Autodesk Fusion 360 part; units mm, degrees
(part 10 of 12)
  line L360 (-90.518, -7.747) -> (-90.518, -11.547)
  line L361 (-94.318, -11.547) -> (-94.318, -7.747)
  line L362 (-90.518, -11.547) -> (-94.318, -11.547)
  line L363 (-94.318, -7.747) -> (-90.518, -7.747)
  arc A1946 (-90.5461, -4.953) -> (-94.5339, -4.953) centre (-92.54, -4.953) ccw
  arc A1947 (-94.5339, -4.953) -> (-90.5461, -4.953) centre (-92.54, -4.953) ccw
  arc A1948 (-88.3109, -5.08) -> (-86.6091, -5.08) centre (-87.46, -5.08) ccw
  arc A1949 (-86.6091, -5.08) -> (-88.3109, -5.08) centre (-87.46, -5.08) ccw
  arc A1950 (-96.7691, -5.08) -> (-98.4709, -5.08) centre (-97.62, -5.08) ccw
  arc A1951 (-98.4709, -5.08) -> (-96.7691, -5.08) centre (-97.62, -5.08) ccw
  line L364 (-60.518, -11.547) -> (-64.318, -11.547)
  line L365 (-64.318, -7.747) -> (-60.518, -7.747)
  line L366 (-60.518, -7.747) -> (-60.518, -11.547)
  line L367 (-64.318, -11.547) -> (-64.318, -7.747)
  arc A1952 (-64.5339, -4.953) -> (-60.5461, -4.953) centre (-62.54, -4.953) ccw
  arc A1953 (-60.5461, -4.953) -> (-64.5339, -4.953) centre (-62.54, -4.953) ccw
  arc A1954 (-56.6091, -5.08) -> (-58.3109, -5.08) centre (-57.46, -5.08) ccw
  arc A1955 (-58.3109, -5.08) -> (-56.6091, -5.08) centre (-57.46, -5.08) ccw
  arc A1956 (-66.7691, -5.08) -> (-68.4709, -5.08) centre (-67.62, -5.08) ccw
  arc A1957 (-68.4709, -5.08) -> (-66.7691, -5.08) centre (-67.62, -5.08) ccw
  line L368 (-34.318, -7.747) -> (-30.518, -7.747)
  line L369 (-30.518, -11.547) -> (-34.318, -11.547)
  line L370 (-30.518, -7.747) -> (-30.518, -11.547)
  line L371 (-34.318, -11.547) -> (-34.318, -7.747)
  arc A1958 (-30.5461, -4.953) -> (-34.5339, -4.953) centre (-32.54, -4.953) ccw
  arc A1959 (-34.5339, -4.953) -> (-30.5461, -4.953) centre (-32.54, -4.953) ccw
  arc A1960 (-26.6091, -5.08) -> (-28.3109, -5.08) centre (-27.46, -5.08) ccw
  arc A1961 (-28.3109, -5.08) -> (-26.6091, -5.08) centre (-27.46, -5.08) ccw
  arc A1962 (-36.7691, -5.08) -> (-38.4709, -5.08) centre (-37.62, -5.08) ccw
  arc A1963 (-38.4709, -5.08) -> (-36.7691, -5.08) centre (-37.62, -5.08) ccw
  line L372 (10.033, -11.801) -> (10.033, -8.001)
  line L373 (13.833, -11.801) -> (10.033, -11.801)
  line L374 (13.833, -8.001) -> (13.833, -11.801)
  line L375 (10.033, -8.001) -> (13.833, -8.001)
  arc A1964 (9.8171, -5.207) -> (13.8049, -5.207) centre (11.811, -5.207) ccw
  arc A1965 (13.8049, -5.207) -> (9.8171, -5.207) centre (11.811, -5.207) ccw
  arc A1966 (17.7419, -5.334) -> (16.0401, -5.334) centre (16.891, -5.334) ccw
  arc A1967 (16.0401, -5.334) -> (17.7419, -5.334) centre (16.891, -5.334) ccw
  arc A1968 (7.5819, -5.334) -> (5.8801, -5.334) centre (6.731, -5.334) ccw
  arc A1969 (5.8801, -5.334) -> (7.5819, -5.334) centre (6.731, -5.334) ccw
  line L376 (49.1491, -12.055) -> (49.1491, -8.255)
  line L377 (49.1491, -8.255) -> (52.9491, -8.255)
  line L378 (52.9491, -8.255) -> (52.9491, -12.055)
  line L379 (52.9491, -12.055) -> (49.1491, -12.055)
  arc A1970 (52.921, -5.461) -> (48.9332, -5.461) centre (50.9271, -5.461) ccw
  arc A1971 (48.9332, -5.461) -> (52.921, -5.461) centre (50.9271, -5.461) ccw
  arc A1972 (55.1562, -5.588) -> (56.858, -5.588) centre (56.0071, -5.588) ccw
  arc A1973 (56.858, -5.588) -> (55.1562, -5.588) centre (56.0071, -5.588) ccw
  arc A1974 (46.698, -5.588) -> (44.9962, -5.588) centre (45.8471, -5.588) ccw
  arc A1975 (44.9962, -5.588) -> (46.698, -5.588) centre (45.8471, -5.588) ccw
  line L380 (-196.538, -36.3221) -> (-192.738, -36.3221)
  line L381 (-192.738, -36.3221) -> (-192.738, -40.1221)
  line L382 (-196.538, -40.1221) -> (-196.538, -36.3221)
  line L383 (-192.738, -40.1221) -> (-196.538, -40.1221)
  arc A1976 (-192.7661, -33.5281) -> (-196.7539, -33.5281) centre (-194.76, -33.5281) ccw
  arc A1977 (-196.7539, -33.5281) -> (-192.7661, -33.5281) centre (-194.76, -33.5281) ccw
  arc A1978 (-188.8291, -33.6551) -> (-190.5309, -33.6551) centre (-189.68, -33.6551) ccw
  arc A1979 (-190.5309, -33.6551) -> (-188.8291, -33.6551) centre (-189.68, -33.6551) ccw
  arc A1980 (-198.9891, -33.6551) -> (-200.6909, -33.6551) centre (-199.84, -33.6551) ccw
  arc A1981 (-200.6909, -33.6551) -> (-198.9891, -33.6551) centre (-199.84, -33.6551) ccw
  line L384 (-162.738, -36.3221) -> (-162.738, -40.1221)
  line L385 (-166.538, -36.3221) -> (-162.738, -36.3221)
  line L386 (-162.738, -40.1221) -> (-166.538, -40.1221)
  line L387 (-166.538, -40.1221) -> (-166.538, -36.3221)
  arc A1982 (-162.7661, -33.5281) -> (-166.7539, -33.5281) centre (-164.76, -33.5281) ccw
  arc A1983 (-166.7539, -33.5281) -> (-162.7661, -33.5281) centre (-164.76, -33.5281) ccw
  arc A1984 (-158.8291, -33.6551) -> (-160.5309, -33.6551) centre (-159.68, -33.6551) ccw
  arc A1985 (-160.5309, -33.6551) -> (-158.8291, -33.6551) centre (-159.68, -33.6551) ccw
  arc A1986 (-168.9891, -33.6551) -> (-170.6909, -33.6551) centre (-169.84, -33.6551) ccw
  arc A1987 (-170.6909, -33.6551) -> (-168.9891, -33.6551) centre (-169.84, -33.6551) ccw
  line L388 (-132.738, -40.1221) -> (-136.538, -40.1221)
  line L389 (-136.538, -36.3221) -> (-132.738, -36.3221)
  line L390 (-136.538, -40.1221) -> (-136.538, -36.3221)
  line L391 (-132.738, -36.3221) -> (-132.738, -40.1221)
  arc A1988 (-132.7661, -33.5281) -> (-136.7539, -33.5281) centre (-134.76, -33.5281) ccw
  arc A1989 (-136.7539, -33.5281) -> (-132.7661, -33.5281) centre (-134.76, -33.5281) ccw
  arc A1990 (-128.8291, -33.6551) -> (-130.5309, -33.6551) centre (-129.68, -33.6551) ccw
  arc A1991 (-130.5309, -33.6551) -> (-128.8291, -33.6551) centre (-129.68, -33.6551) ccw
  arc A1992 (-140.6909, -33.6551) -> (-138.9891, -33.6551) centre (-139.84, -33.6551) ccw
  arc A1993 (-138.9891, -33.6551) -> (-140.6909, -33.6551) centre (-139.84, -33.6551) ccw
  line L392 (-102.738, -36.3221) -> (-102.738, -40.1221)
  line L393 (-106.538, -40.1221) -> (-106.538, -36.3221)
  line L394 (-102.738, -40.1221) -> (-106.538, -40.1221)
  line L395 (-106.538, -36.3221) -> (-102.738, -36.3221)
  arc A1994 (-102.7661, -33.5281) -> (-106.7539, -33.5281) centre (-104.76, -33.5281) ccw
  arc A1995 (-106.7539, -33.5281) -> (-102.7661, -33.5281) centre (-104.76, -33.5281) ccw
  arc A1996 (-98.8291, -33.6551) -> (-100.5309, -33.6551) centre (-99.68, -33.6551) ccw
  arc A1997 (-100.5309, -33.6551) -> (-98.8291, -33.6551) centre (-99.68, -33.6551) ccw
  arc A1998 (-108.9891, -33.6551) -> (-110.6909, -33.6551) centre (-109.84, -33.6551) ccw
  arc A1999 (-110.6909, -33.6551) -> (-108.9891, -33.6551) centre (-109.84, -33.6551) ccw
  line L396 (-76.538, -40.1221) -> (-76.538, -36.3221)
  line L397 (-76.538, -36.3221) -> (-72.738, -36.3221)
  line L398 (-72.738, -36.3221) -> (-72.738, -40.1221)
  line L399 (-72.738, -40.1221) -> (-76.538, -40.1221)
  arc A2000 (-76.7539, -33.5281) -> (-72.7661, -33.5281) centre (-74.76, -33.5281) ccw
  arc A2001 (-72.7661, -33.5281) -> (-76.7539, -33.5281) centre (-74.76, -33.5281) ccw
  arc A2002 (-68.8291, -33.6551) -> (-70.5309, -33.6551) centre (-69.68, -33.6551) ccw
  arc A2003 (-70.5309, -33.6551) -> (-68.8291, -33.6551) centre (-69.68, -33.6551) ccw
  arc A2004 (-80.6909, -33.6551) -> (-78.9891, -33.6551) centre (-79.84, -33.6551) ccw
  arc A2005 (-78.9891, -33.6551) -> (-80.6909, -33.6551) centre (-79.84, -33.6551) ccw
  line L400 (-42.738, -40.1221) -> (-46.538, -40.1221)
  line L401 (-46.538, -36.3221) -> (-42.738, -36.3221)
  line L402 (-42.738, -36.3221) -> (-42.738, -40.1221)
  line L403 (-46.538, -40.1221) -> (-46.538, -36.3221)
  arc A2006 (-46.7539, -33.5281) -> (-42.7661, -33.5281) centre (-44.76, -33.5281) ccw
  arc A2007 (-42.7661, -33.5281) -> (-46.7539, -33.5281) centre (-44.76, -33.5281) ccw
  arc A2008 (-40.5309, -33.6551) -> (-38.8291, -33.6551) centre (-39.68, -33.6551) ccw
  arc A2009 (-38.8291, -33.6551) -> (-40.5309, -33.6551) centre (-39.68, -33.6551) ccw
  arc A2010 (-48.9891, -33.6551) -> (-50.6909, -33.6551) centre (-49.84, -33.6551) ccw
  arc A2011 (-50.6909, -33.6551) -> (-48.9891, -33.6551) centre (-49.84, -33.6551) ccw
  line L404 (-12.738, -40.1221) -> (-16.538, -40.1221)
  line L405 (-12.738, -36.3221) -> (-12.738, -40.1221)
  line L406 (-16.538, -40.1221) -> (-16.538, -36.3221)
  line L407 (-16.538, -36.3221) -> (-12.738, -36.3221)
  arc A2012 (-16.7539, -33.5281) -> (-12.7661, -33.5281) centre (-14.76, -33.5281) ccw
  arc A2013 (-12.7661, -33.5281) -> (-16.7539, -33.5281) centre (-14.76, -33.5281) ccw
  line L408 (-12.7661, -33.5281) -> (-12.7661, -33.5281)
  arc A2014 (-8.8291, -33.6551) -> (-10.5309, -33.6551) centre (-9.68, -33.6551) ccw
  arc A2015 (-10.5309, -33.6551) -> (-8.8291, -33.6551) centre (-9.68, -33.6551) ccw
  arc A2016 (-20.6909, -33.6551) -> (-18.9891, -33.6551) centre (-19.84, -33.6551) ccw
  arc A2017 (-18.9891, -33.6551) -> (-20.6909, -33.6551) centre (-19.84, -33.6551) ccw
  line L409 (17.262, -36.3221) -> (17.262, -40.1221)
  line L410 (13.462, -36.3221) -> (17.262, -36.3221)
  line L411 (13.462, -40.1221) -> (13.462, -36.3221)
  line L412 (17.262, -40.1221) -> (13.462, -40.1221)
  arc A2018 (13.2461, -33.5281) -> (17.2339, -33.5281) centre (15.24, -33.5281) ccw
  arc A2019 (17.2339, -33.5281) -> (13.2461, -33.5281) centre (15.24, -33.5281) ccw
  line L413 (17.2339, -33.5281) -> (17.2339, -33.5281)
  arc A2020 (21.1709, -33.6551) -> (19.4691, -33.6551) centre (20.32, -33.6551) ccw
  arc A2021 (19.4691, -33.6551) -> (21.1709, -33.6551) centre (20.32, -33.6551) ccw
  arc A2022 (11.0109, -33.6551) -> (9.3091, -33.6551) centre (10.16, -33.6551) ccw
  arc A2023 (9.3091, -33.6551) -> (11.0109, -33.6551) centre (10.16, -33.6551) ccw
  line L414 (49.1466, -41.1381) -> (49.1466, -37.3381)
  line L415 (52.9466, -37.3381) -> (52.9466, -41.1381)
  line L416 (49.1466, -37.3381) -> (52.9466, -37.3381)
  line L417 (52.9466, -41.1381) -> (49.1466, -41.1381)
  arc A2024 (48.9307, -34.5441) -> (52.9185, -34.5441) centre (50.9246, -34.5441) ccw
  arc A2025 (52.9185, -34.5441) -> (48.9307, -34.5441) centre (50.9246, -34.5441) ccw
  arc A2026 (56.8555, -34.6711) -> (55.1537, -34.6711) centre (56.0046, -34.6711) ccw
  arc A2027 (55.1537, -34.6711) -> (56.8555, -34.6711) centre (56.0046, -34.6711) ccw
  arc A2028 (44.9937, -34.6711) -> (46.6955, -34.6711) centre (45.8446, -34.6711) ccw
  arc A2029 (46.6955, -34.6711) -> (44.9937, -34.6711) centre (45.8446, -34.6711) ccw
  line L418 (-185.9511, -63.3791) -> (-185.9511, -67.1791)
  line L419 (-185.9511, -67.1791) -> (-189.7511, -67.1791)
  line L420 (-189.7511, -63.3791) -> (-185.9511, -63.3791)
  line L421 (-189.7511, -67.1791) -> (-189.7511, -63.3791)
  arc A2030 (-189.967, -60.5851) -> (-185.9792, -60.5851) centre (-187.9731, -60.5851) ccw
  arc A2031 (-185.9792, -60.5851) -> (-189.967, -60.5851) centre (-187.9731, -60.5851) ccw
  arc A2032 (-182.0422, -60.7121) -> (-183.744, -60.7121) centre (-182.8931, -60.7121) ccw
  arc A2033 (-183.744, -60.7121) -> (-182.0422, -60.7121) centre (-182.8931, -60.7121) ccw
  arc A2034 (-192.2022, -60.7121) -> (-193.904, -60.7121) centre (-193.0531, -60.7121) ccw
  arc A2035 (-193.904, -60.7121) -> (-192.2022, -60.7121) centre (-193.0531, -60.7121) ccw
  line L422 (-155.9511, -67.1791) -> (-159.7511, -67.1791)
  line L423 (-155.9511, -63.3791) -> (-155.9511, -67.1791)
  line L424 (-159.7511, -63.3791) -> (-155.9511, -63.3791)
  line L425 (-159.7511, -67.1791) -> (-159.7511, -63.3791)
  arc A2036 (-155.9792, -60.5851) -> (-159.967, -60.5851) centre (-157.9731, -60.5851) ccw
  arc A2037 (-159.967, -60.5851) -> (-155.9792, -60.5851) centre (-157.9731, -60.5851) ccw
  arc A2038 (-152.0422, -60.7121) -> (-153.744, -60.7121) centre (-152.8931, -60.7121) ccw
  arc A2039 (-153.744, -60.7121) -> (-152.0422, -60.7121) centre (-152.8931, -60.7121) ccw
  arc A2040 (-162.2022, -60.7121) -> (-163.904, -60.7121) centre (-163.0531, -60.7121) ccw
  arc A2041 (-163.904, -60.7121) -> (-162.2022, -60.7121) centre (-163.0531, -60.7121) ccw
  line L426 (-129.7511, -67.1791) -> (-129.7511, -63.3791)
  line L427 (-125.9511, -63.3791) -> (-125.9511, -67.1791)
  line L428 (-125.9511, -67.1791) -> (-129.7511, -67.1791)
  line L429 (-129.7511, -63.3791) -> (-125.9511, -63.3791)
  arc A2042 (-129.967, -60.5851) -> (-125.9792, -60.5851) centre (-127.9731, -60.5851) ccw
  arc A2043 (-125.9792, -60.5851) -> (-129.967, -60.5851) centre (-127.9731, -60.5851) ccw
  arc A2044 (-123.744, -60.7121) -> (-122.0422, -60.7121) centre (-122.8931, -60.7121) ccw
  arc A2045 (-122.0422, -60.7121) -> (-123.744, -60.7121) centre (-122.8931, -60.7121) ccw
  arc A2046 (-133.904, -60.7121) -> (-132.2022, -60.7121) centre (-133.0531, -60.7121) ccw
  arc A2047 (-132.2022, -60.7121) -> (-133.904, -60.7121) centre (-133.0531, -60.7121) ccw
  line L430 (-95.9511, -67.1791) -> (-99.7511, -67.1791)
  line L431 (-99.7511, -67.1791) -> (-99.7511, -63.3791)
  line L432 (-95.9511, -63.3791) -> (-95.9511, -67.1791)
  line L433 (-99.7511, -63.3791) -> (-95.9511, -63.3791)
  arc A2048 (-95.9792, -60.5851) -> (-99.967, -60.5851) centre (-97.9731, -60.5851) ccw
  arc A2049 (-99.967, -60.5851) -> (-95.9792, -60.5851) centre (-97.9731, -60.5851) ccw
  arc A2050 (-93.744, -60.7121) -> (-92.0422, -60.7121) centre (-92.8931, -60.7121) ccw
  arc A2051 (-92.0422, -60.7121) -> (-93.744, -60.7121) centre (-92.8931, -60.7121) ccw
  arc A2052 (-103.904, -60.7121) -> (-102.2022, -60.7121) centre (-103.0531, -60.7121) ccw
  arc A2053 (-102.2022, -60.7121) -> (-103.904, -60.7121) centre (-103.0531, -60.7121) ccw
  line L434 (-65.9511, -63.3791) -> (-65.9511, -67.1791)
  line L435 (-65.9511, -67.1791) -> (-69.7511, -67.1791)
  line L436 (-69.7511, -67.1791) -> (-69.7511, -63.3791)
  line L437 (-69.7511, -63.3791) -> (-65.9511, -63.3791)
  arc A2054 (-65.9792, -60.5851) -> (-69.967, -60.5851) centre (-67.9731, -60.5851) ccw
  arc A2055 (-69.967, -60.5851) -> (-65.9792, -60.5851) centre (-67.9731, -60.5851) ccw
  arc A2056 (-63.744, -60.7121) -> (-62.0422, -60.7121) centre (-62.8931, -60.7121) ccw
  arc A2057 (-62.0422, -60.7121) -> (-63.744, -60.7121) centre (-62.8931, -60.7121) ccw
  arc A2058 (-73.904, -60.7121) -> (-72.2022, -60.7121) centre (-73.0531, -60.7121) ccw
  arc A2059 (-72.2022, -60.7121) -> (-73.904, -60.7121) centre (-73.0531, -60.7121) ccw
  line L438 (-39.7511, -63.3791) -> (-35.9511, -63.3791)
  line L439 (-35.9511, -67.1791) -> (-39.7511, -67.1791)
  line L440 (-39.7511, -67.1791) -> (-39.7511, -63.3791)
  line L441 (-35.9511, -63.3791) -> (-35.9511, -67.1791)
  arc A2060 (-35.9792, -60.5851) -> (-39.967, -60.5851) centre (-37.9731, -60.5851) ccw
  arc A2061 (-39.967, -60.5851) -> (-35.9792, -60.5851) centre (-37.9731, -60.5851) ccw
  arc A2062 (-33.744, -60.7121) -> (-32.0422, -60.7121) centre (-32.8931, -60.7121) ccw
  arc A2063 (-32.0422, -60.7121) -> (-33.744, -60.7121) centre (-32.8931, -60.7121) ccw
  arc A2064 (-43.904, -60.7121) -> (-42.2022, -60.7121) centre (-43.0531, -60.7121) ccw
  arc A2065 (-42.2022, -60.7121) -> (-43.904, -60.7121) centre (-43.0531, -60.7121) ccw
  line L442 (3.175, -68.1891) -> (3.175, -64.3891)
  line L443 (6.975, -68.1891) -> (3.175, -68.1891)
  line L444 (6.975, -64.3891) -> (6.975, -68.1891)
  line L445 (3.175, -64.3891) -> (6.975, -64.3891)
  arc A2066 (6.9469, -61.5951) -> (2.9591, -61.5951) centre (4.953, -61.5951) ccw
  arc A2067 (2.9591, -61.5951) -> (6.9469, -61.5951) centre (4.953, -61.5951) ccw
  arc A2068 (9.1821, -61.7221) -> (10.8839, -61.7221) centre (10.033, -61.7221) ccw
  arc A2069 (10.8839, -61.7221) -> (9.1821, -61.7221) centre (10.033, -61.7221) ccw
  arc A2070 (0.7239, -61.7221) -> (-0.9779, -61.7221) centre (-0.127, -61.7221) ccw
  arc A2071 (-0.9779, -61.7221) -> (0.7239, -61.7221) centre (-0.127, -61.7221) ccw
  line L446 (-178.4989, -94.4882) -> (-174.6989, -94.4882)
  line L447 (-174.6989, -98.2882) -> (-178.4989, -98.2882)
  line L448 (-178.4989, -98.2882) -> (-178.4989, -94.4882)
  line L449 (-174.6989, -94.4882) -> (-174.6989, -98.2882)
  arc A2072 (-174.7269, -91.6942) -> (-178.7148, -91.6942) centre (-176.7209, -91.6942) ccw
  arc A2073 (-178.7148, -91.6942) -> (-174.7269, -91.6942) centre (-176.7209, -91.6942) ccw
  arc A2074 (-172.4917, -91.8212) -> (-170.7899, -91.8212) centre (-171.6408, -91.8212) ccw
  arc A2075 (-170.7899, -91.8212) -> (-172.4917, -91.8212) centre (-171.6408, -91.8212) ccw
  arc A2076 (-180.95, -91.8212) -> (-182.6518, -91.8212) centre (-181.8009, -91.8212) ccw
  arc A2077 (-182.6518, -91.8212) -> (-180.95, -91.8212) centre (-181.8009, -91.8212) ccw
  line L450 (55.8701, -71.7551) -> (55.8701, -75.5551)
  line L451 (52.0701, -75.5551) -> (52.0701, -71.7551)
  line L452 (52.0701, -71.7551) -> (55.8701, -71.7551)
  line L453 (55.8701, -75.5551) -> (52.0701, -75.5551)
  arc A2078 (51.8542, -68.9611) -> (55.842, -68.9611) centre (53.8481, -68.9611) ccw
  arc A2079 (55.842, -68.9611) -> (51.8542, -68.9611) centre (53.8481, -68.9611) ccw
  arc A2080 (58.0772, -69.0881) -> (59.779, -69.0881) centre (58.9281, -69.0881) ccw
  arc A2081 (59.779, -69.0881) -> (58.0772, -69.0881) centre (58.9281, -69.0881) ccw
  arc A2082 (47.9172, -69.0881) -> (49.619, -69.0881) centre (48.7681, -69.0881) ccw
  arc A2083 (49.619, -69.0881) -> (47.9172, -69.0881) centre (48.7681, -69.0881) ccw
  line L454 (-144.2823, -94.4882) -> (-144.2823, -98.2882)
  line L455 (-148.0823, -98.2882) -> (-148.0823, -94.4882)
  line L456 (-148.0823, -94.4882) -> (-144.2823, -94.4882)
  line L457 (-144.2823, -98.2882) -> (-148.0823, -98.2882)
  arc A2084 (-144.3104, -91.6942) -> (-148.2982, -91.6942) centre (-146.3043, -91.6942) ccw
  arc A2085 (-148.2982, -91.6942) -> (-144.3104, -91.6942) centre (-146.3043, -91.6942) ccw
  arc A2086 (-140.3734, -91.8212) -> (-142.0752, -91.8212) centre (-141.2243, -91.8212) ccw
  arc A2087 (-142.0752, -91.8212) -> (-140.3734, -91.8212) centre (-141.2243, -91.8212) ccw
  arc A2088 (-150.5335, -91.8212) -> (-152.2353, -91.8212) centre (-151.3844, -91.8212) ccw
  arc A2089 (-152.2353, -91.8212) -> (-150.5335, -91.8212) centre (-151.3844, -91.8212) ccw
  line L458 (-117.6658, -98.2882) -> (-117.6658, -94.4882)
  line L459 (-113.8658, -94.4882) -> (-113.8658, -98.2882)
  line L460 (-113.8658, -98.2882) -> (-117.6658, -98.2882)
  line L461 (-117.6658, -94.4882) -> (-113.8658, -94.4882)
  arc A2090 (-113.8939, -91.6942) -> (-117.8817, -91.6942) centre (-115.8878, -91.6942) ccw
  arc A2091 (-117.8817, -91.6942) -> (-113.8939, -91.6942) centre (-115.8878, -91.6942) ccw
  arc A2092 (-111.6587, -91.8212) -> (-109.9569, -91.8212) centre (-110.8078, -91.8212) ccw
  arc A2093 (-109.9569, -91.8212) -> (-111.6587, -91.8212) centre (-110.8078, -91.8212) ccw
  arc A2094 (-120.1169, -91.8212) -> (-121.8187, -91.8212) centre (-120.9678, -91.8212) ccw
  arc A2095 (-121.8187, -91.8212) -> (-120.1169, -91.8212) centre (-120.9678, -91.8212) ccw
  line L462 (-87.2492, -98.2882) -> (-87.2492, -94.4882)
  line L463 (-83.4492, -94.4882) -> (-83.4492, -98.2882)
  line L464 (-83.4492, -98.2882) -> (-87.2492, -98.2882)
  line L465 (-87.2492, -94.4882) -> (-83.4492, -94.4882)
  arc A2096 (-87.4651, -91.6942) -> (-83.4773, -91.6942) centre (-85.4712, -91.6942) ccw
  arc A2097 (-83.4773, -91.6942) -> (-87.4651, -91.6942) centre (-85.4712, -91.6942) ccw
  arc A2098 (-79.5403, -91.8212) -> (-81.2421, -91.8212) centre (-80.3912, -91.8212) ccw
  arc A2099 (-81.2421, -91.8212) -> (-79.5403, -91.8212) centre (-80.3912, -91.8212) ccw
  arc A2100 (-91.4021, -91.8212) -> (-89.7003, -91.8212) centre (-90.5512, -91.8212) ccw
  arc A2101 (-89.7003, -91.8212) -> (-91.4021, -91.8212) centre (-90.5512, -91.8212) ccw
  line L466 (-53.0326, -94.4882) -> (-53.0326, -98.2882)
  line L467 (-56.8326, -94.4882) -> (-53.0326, -94.4882)
  line L468 (-56.8326, -98.2882) -> (-56.8326, -94.4882)
  line L469 (-53.0326, -98.2882) -> (-56.8326, -98.2882)
  arc A2102 (-53.0607, -91.6942) -> (-57.0485, -91.6942) centre (-55.0546, -91.6942) ccw
  arc A2103 (-57.0485, -91.6942) -> (-53.0607, -91.6942) centre (-55.0546, -91.6942) ccw
  arc A2104 (-50.8255, -91.8212) -> (-49.1237, -91.8212) centre (-49.9746, -91.8212) ccw
  arc A2105 (-49.1237, -91.8212) -> (-50.8255, -91.8212) centre (-49.9746, -91.8212) ccw
  arc A2106 (-60.9855, -91.8212) -> (-59.2837, -91.8212) centre (-60.1346, -91.8212) ccw
  arc A2107 (-59.2837, -91.8212) -> (-60.9855, -91.8212) centre (-60.1346, -91.8212) ccw
  line L470 (-22.6161, -94.4882) -> (-22.6161, -98.2882)
  line L471 (-26.4161, -94.4882) -> (-22.6161, -94.4882)
  line L472 (-26.4161, -98.2882) -> (-26.4161, -94.4882)
  line L473 (-22.6161, -98.2882) -> (-26.4161, -98.2882)
  arc A2108 (-26.632, -91.6942) -> (-22.6441, -91.6942) centre (-24.638, -91.6942) ccw
  arc A2109 (-22.6441, -91.6942) -> (-26.632, -91.6942) centre (-24.638, -91.6942) ccw
  arc A2110 (-18.7071, -91.8212) -> (-20.4089, -91.8212) centre (-19.558, -91.8212) ccw
  arc A2111 (-20.4089, -91.8212) -> (-18.7071, -91.8212) centre (-19.558, -91.8212) ccw
  arc A2112 (-30.569, -91.8212) -> (-28.8672, -91.8212) centre (-29.7181, -91.8212) ccw
  arc A2113 (-28.8672, -91.8212) -> (-30.569, -91.8212) centre (-29.7181, -91.8212) ccw
  line L474 (3.937, -94.5894) -> (7.737, -94.5894)
  line L475 (3.937, -98.3894) -> (3.937, -94.5894)
  line L476 (7.737, -98.3894) -> (3.937, -98.3894)
  line L477 (7.737, -94.5894) -> (7.737, -98.3894)
  arc A2114 (7.7089, -91.7954) -> (3.7211, -91.7954) centre (5.715, -91.7954) ccw
  arc A2115 (3.7211, -91.7954) -> (7.7089, -91.7954) centre (5.715, -91.7954) ccw
  arc A2116 (11.6459, -91.9224) -> (9.9441, -91.9224) centre (10.795, -91.9224) ccw
  arc A2117 (9.9441, -91.9224) -> (11.6459, -91.9224) centre (10.795, -91.9224) ccw
  arc A2118 (-0.2159, -91.9224) -> (1.4859, -91.9224) centre (0.635, -91.9224) ccw
  arc A2119 (1.4859, -91.9224) -> (-0.2159, -91.9224) centre (0.635, -91.9224) ccw
  line L478 (-159.0293, -128.7242) -> (-159.0293, -124.9242)
  line L479 (-155.2293, -124.9242) -> (-155.2293, -128.7242)
  line L480 (-159.0293, -124.9242) -> (-155.2293, -124.9242)
  line L481 (-155.2293, -128.7242) -> (-159.0293, -128.7242)
  arc A2120 (-159.2452, -122.1302) -> (-155.2574, -122.1302) centre (-157.2513, -122.1302) ccw
  arc A2121 (-155.2574, -122.1302) -> (-159.2452, -122.1302) centre (-157.2513, -122.1302) ccw
  arc A2122 (-153.0222, -122.2572) -> (-151.3204, -122.2572) centre (-152.1713, -122.2572) ccw
  arc A2123 (-151.3204, -122.2572) -> (-153.0222, -122.2572) centre (-152.1713, -122.2572) ccw
  arc A2124 (-163.1822, -122.2572) -> (-161.4804, -122.2572) centre (-162.3313, -122.2572) ccw
  arc A2125 (-161.4804, -122.2572) -> (-163.1822, -122.2572) centre (-162.3313, -122.2572) ccw
  line L482 (-112.57, -128.7242) -> (-116.37, -128.7242)
  line L483 (-112.57, -124.9242) -> (-112.57, -128.7242)
  line L484 (-116.37, -124.9242) -> (-112.57, -124.9242)
  line L485 (-116.37, -128.7242) -> (-116.37, -124.9242)
  arc A2126 (-112.598, -122.1302) -> (-116.5859, -122.1302) centre (-114.5919, -122.1302) ccw
  arc A2127 (-116.5859, -122.1302) -> (-112.598, -122.1302) centre (-114.5919, -122.1302) ccw
  arc A2128 (-110.3628, -122.2572) -> (-108.661, -122.2572) centre (-109.5119, -122.2572) ccw
  arc A2129 (-108.661, -122.2572) -> (-110.3628, -122.2572) centre (-109.5119, -122.2572) ccw
  arc A2130 (-120.5229, -122.2572) -> (-118.8211, -122.2572) centre (-119.672, -122.2572) ccw
  arc A2131 (-118.8211, -122.2572) -> (-120.5229, -122.2572) centre (-119.672, -122.2572) ccw
  line L486 (-86.37, -128.7242) -> (-86.37, -124.9242)
  line L487 (-82.57, -128.7242) -> (-86.37, -128.7242)
  line L488 (-82.57, -124.9242) -> (-82.57, -128.7242)
  line L489 (-86.37, -124.9242) -> (-82.57, -124.9242)
  arc A2132 (-82.598, -122.1302) -> (-86.5859, -122.1302) centre (-84.5919, -122.1302) ccw
  arc A2133 (-86.5859, -122.1302) -> (-82.598, -122.1302) centre (-84.5919, -122.1302) ccw
  arc A2134 (-80.3628, -122.2572) -> (-78.661, -122.2572) centre (-79.5119, -122.2572) ccw
  arc A2135 (-78.661, -122.2572) -> (-80.3628, -122.2572) centre (-79.5119, -122.2572) ccw
  arc A2136 (-88.8211, -122.2572) -> (-90.5229, -122.2572) centre (-89.672, -122.2572) ccw
  arc A2137 (-90.5229, -122.2572) -> (-88.8211, -122.2572) centre (-89.672, -122.2572) ccw
  line L490 (-56.37, -128.7242) -> (-56.37, -124.9242)
  line L491 (-56.37, -124.9242) -> (-52.57, -124.9242)
  line L492 (-52.57, -128.7242) -> (-56.37, -128.7242)
  line L493 (-52.57, -124.9242) -> (-52.57, -128.7242)
  arc A2138 (-56.5859, -122.1302) -> (-52.598, -122.1302) centre (-54.5919, -122.1302) ccw
  arc A2139 (-52.598, -122.1302) -> (-56.5859, -122.1302) centre (-54.5919, -122.1302) ccw
  arc A2140 (-48.661, -122.2572) -> (-50.3628, -122.2572) centre (-49.5119, -122.2572) ccw
  arc A2141 (-50.3628, -122.2572) -> (-48.661, -122.2572) centre (-49.5119, -122.2572) ccw
  arc A2142 (-60.5229, -122.2572) -> (-58.8211, -122.2572) centre (-59.672, -122.2572) ccw
  arc A2143 (-58.8211, -122.2572) -> (-60.5229, -122.2572) centre (-59.672, -122.2572) ccw
  line L494 (-22.57, -124.9242) -> (-22.57, -128.7242)
  line L495 (-26.37, -124.9242) -> (-22.57, -124.9242)
  line L496 (-22.57, -128.7242) -> (-26.37, -128.7242)
  line L497 (-26.37, -128.7242) -> (-26.37, -124.9242)
  arc A2144 (-26.5859, -122.1302) -> (-22.598, -122.1302) centre (-24.5919, -122.1302) ccw
  arc A2145 (-22.598, -122.1302) -> (-26.5859, -122.1302) centre (-24.5919, -122.1302) ccw
  arc A2146 (-20.3628, -122.2572) -> (-18.661, -122.2572) centre (-19.5119, -122.2572) ccw
  arc A2147 (-18.661, -122.2572) -> (-20.3628, -122.2572) centre (-19.5119, -122.2572) ccw
  arc A2148 (-30.5229, -122.2572) -> (-28.8211, -122.2572) centre (-29.672, -122.2572) ccw
  arc A2149 (-28.8211, -122.2572) -> (-30.5229, -122.2572) centre (-29.672, -122.2572) ccw
  line L498 (3.63, -124.9242) -> (7.43, -124.9242)
  line L499 (7.43, -124.9242) -> (7.43, -128.7242)
  line L500 (7.43, -128.7242) -> (3.63, -128.7242)
  line L501 (3.63, -128.7242) -> (3.63, -124.9242)
  arc A2150 (3.4141, -122.1302) -> (7.402, -122.1302) centre (5.4081, -122.1302) ccw
  line L502 (7.402, -122.1302) -> (7.402, -122.1302)
  arc A2151 (7.402, -122.1302) -> (3.4141, -122.1302) centre (5.4081, -122.1302) ccw
  arc A2152 (11.339, -122.2572) -> (9.6372, -122.2572) centre (10.4881, -122.2572) ccw
  arc A2153 (9.6372, -122.2572) -> (11.339, -122.2572) centre (10.4881, -122.2572) ccw
  arc A2154 (-0.5229, -122.2572) -> (1.1789, -122.2572) centre (0.328, -122.2572) ccw
  arc A2155 (1.1789, -122.2572) -> (-0.5229, -122.2572) centre (0.328, -122.2572) ccw
  line L503 (37.43, -124.9242) -> (37.43, -128.7242)
  line L504 (33.63, -124.9242) -> (37.43, -124.9242)
  line L505 (37.43, -128.7242) -> (33.63, -128.7242)
  line L506 (33.63, -128.7242) -> (33.63, -124.9242)
  arc A2156 (37.402, -122.1302) -> (33.4141, -122.1302) centre (35.4081, -122.1302) ccw
  arc A2157 (33.4141, -122.1302) -> (37.402, -122.1302) centre (35.4081, -122.1302) ccw
  arc A2158 (39.6372, -122.2572) -> (41.339, -122.2572) centre (40.4881, -122.2572) ccw
  arc A2159 (41.339, -122.2572) -> (39.6372, -122.2572) centre (40.4881, -122.2572) ccw
  arc A2160 (31.1789, -122.2572) -> (29.4771, -122.2572) centre (30.328, -122.2572) ccw
  arc A2161 (29.4771, -122.2572) -> (31.1789, -122.2572) centre (30.328, -122.2572) ccw
  arc A2162 (-167.4186, 33.9116) -> (-168.9187, 33.9116) centre (-168.1687, 33.9116) ccw
  arc A2163 (-168.9187, 33.9116) -> (-167.4186, 33.9116) centre (-168.1687, 33.9116) ccw
  arc A2164 (-167.3678, 26.8936) -> (-168.8679, 26.8936) centre (-168.1179, 26.8936) ccw
  arc A2165 (-168.8679, 26.8936) -> (-167.3678, 26.8936) centre (-168.1179, 26.8936) ccw
  line L507 (94.3024, -53.4357) -> (94.2008, -53.4865)
  line L508 (94.6047, -54.0402) -> (94.8561, -54.0402)
  line L509 (94.15, -53.738) -> (94.2008, -53.8878)
  line L510 (94.2008, -53.8878) -> (94.3532, -53.9894)
  line L511 (95.1584, -53.5373) -> (95.0593, -53.4357)
  line L512 (94.7063, -53.4357) -> (94.6047, -53.5373)
  line L513 (94.6047, -53.5373) -> (94.5539, -53.6872)
  line L514 (95.0593, -53.4357) -> (94.9069, -53.3849)
  line L515 (94.7063, -53.9894) -> (94.8561, -54.0402)
  line L516 (95.2092, -53.6872) -> (95.1584, -53.5373)
  line L517 (94.9069, -53.3849) -> (94.8561, -53.3849)
  line L518 (94.8561, -53.3849) -> (94.7063, -53.4357)
  line L519 (94.5539, -53.738) -> (94.6047, -53.8878)
  line L520 (94.5539, -53.6872) -> (94.5539, -53.738)
  line L521 (94.6047, -53.8878) -> (94.7063, -53.9894)
  line L522 (95.1584, -53.8878) -> (95.2092, -53.738)
  line L523 (95.2092, -53.738) -> (95.2092, -53.6872)
  line L524 (95.0593, -53.9894) -> (95.1584, -53.8878)
  line L525 (94.8561, -54.0402) -> (95.0593, -53.9894)
  line L526 (94.15, -53.6364) -> (94.15, -53.738)
  line L527 (94.2008, -53.4865) -> (94.15, -53.6364)
  line L528 (94.3532, -53.9894) -> (94.6047, -54.0402)
  line L529 (94.5539, -52.5366) -> (94.5031, -52.4375)
  line L530 (94.6047, -52.7398) -> (94.5539, -52.5366)
  line L531 (94.6047, -52.6382) -> (94.6555, -52.4858)
  line L532 (95.2092, -52.5874) -> (95.2092, -52.7906)
  line L533 (94.15, -52.7906) -> (94.2008, -52.9404)
  line L534 (95.1584, -52.4375) -> (95.2092, -52.5874)
  line L535 (94.404, -52.9912) -> (94.5031, -52.9404)
  line L536 (95.1076, -52.9912) -> (95.0085, -53.042)
  line L537 (95.1584, -52.9404) -> (95.1076, -52.9912)
  line L538 (94.3024, -52.9912) -> (94.404, -52.9912)
  line L539 (94.8561, -52.3359) -> (95.0085, -52.3359)
  line L540 (94.2008, -52.9404) -> (94.3024, -52.9912)
  line L541 (95.0085, -53.042) -> (94.8561, -53.042)
  line L542 (94.7571, -52.3867) -> (94.8561, -52.3359)
  line L543 (95.1076, -52.3867) -> (95.1584, -52.4375)
  line L544 (94.6555, -52.4858) -> (94.7571, -52.3867)
  line L545 (94.2008, -52.4375) -> (94.15, -52.5874)
  line L546 (94.15, -52.5874) -> (94.15, -52.7906)
  line L547 (94.8561, -53.042) -> (94.7571, -52.9912)
  line L548 (95.0085, -52.3359) -> (95.1076, -52.3867)
  line L549 (94.5031, -52.9404) -> (94.5539, -52.8388)
  line L550 (94.5539, -52.8388) -> (94.6047, -52.6382)
  line L551 (94.5031, -52.4375) -> (94.404, -52.3867)
  line L552 (94.7571, -52.9912) -> (94.6555, -52.8896)
  line L553 (94.3024, -52.3867) -> (94.2008, -52.4375)
  line L554 (94.404, -52.3867) -> (94.3024, -52.3867)
  line L555 (94.6555, -52.8896) -> (94.6047, -52.7398)
  line L556 (95.2092, -52.7906) -> (95.1584, -52.9404)
  line L557 (95.2092, -51.5891) -> (95.1584, -51.4367)
  line L558 (94.3532, -51.3377) -> (94.2008, -51.4367)
  line L559 (94.2008, -51.4367) -> (94.15, -51.5891)
  line L560 (95.1584, -51.8406) -> (95.2092, -51.6907)
  line L561 (95.0085, -51.3377) -> (94.7571, -51.2869)
  line L562 (94.15, -51.6907) -> (94.2008, -51.8406)
  line L563 (94.6047, -51.993) -> (94.7571, -51.993)
  line L564 (94.2008, -51.8406) -> (94.3532, -51.9422)
  line L565 (94.7571, -51.2869) -> (94.6047, -51.2869)
  line L566 (94.15, -51.5891) -> (94.15, -51.6907)
  line L567 (95.0085, -51.9422) -> (95.1584, -51.8406)
  line L568 (94.7571, -51.993) -> (95.0085, -51.9422)
  line L569 (94.6047, -51.2869) -> (94.3532, -51.3377)
  line L570 (95.2092, -51.6907) -> (95.2092, -51.5891)
  line L571 (94.3532, -51.9422) -> (94.6047, -51.993)
  line L572 (95.1584, -51.4367) -> (95.0085, -51.3377)
  line L573 (94.5031, -50.2887) -> (94.6555, -50.3395)
  line L574 (95.1584, -50.8424) -> (95.0593, -50.8932)
  line L575 (94.3024, -50.3395) -> (94.5031, -50.2887)
  line L576 (94.15, -50.5909) -> (94.2008, -50.4385)
  line L577 (95.1584, -50.4385) -> (95.2092, -50.5909)
  line L578 (94.4523, -50.944) -> (94.3024, -50.8932)
  line L579 (94.2008, -50.7916) -> (94.15, -50.6417)
  line L580 (94.5031, -50.944) -> (94.4523, -50.944)
  line L581 (94.3024, -50.8932) -> (94.2008, -50.7916)
  line L582 (94.7571, -50.2887) -> (95.0085, -50.3395)
  line L583 (95.2092, -50.5909) -> (95.2092, -50.6925)
  line L584 (94.8053, -50.6417) -> (94.7571, -50.7916)
  line L585 (94.2008, -50.4385) -> (94.3024, -50.3395)
  line L586 (94.7571, -50.7916) -> (94.6555, -50.8932)
  line L587 (94.6555, -50.8932) -> (94.5031, -50.944)
  line L588 (94.7571, -50.4385) -> (94.8053, -50.5909)
  line L589 (94.6555, -50.3395) -> (94.7571, -50.4385)
  line L590 (94.5031, -50.2887) -> (94.7571, -50.2887)
  line L591 (94.15, -50.6417) -> (94.15, -50.5909)
  line L592 (95.2092, -50.6925) -> (95.1584, -50.8424)
  line L593 (94.8053, -50.5909) -> (94.8053, -50.6417)
  line L594 (95.0085, -50.3395) -> (95.1584, -50.4385)
  line L595 (95.0085, -49.8442) -> (94.9577, -49.895)
  line L596 (95.0593, -49.895) -> (95.0085, -49.8442)
  line L597 (94.9577, -49.895) -> (95.0085, -49.9458)
  line L598 (95.0085, -49.9458) -> (95.0593, -49.895)
  line L599 (94.3024, -48.8459) -> (94.2008, -48.8967)
  line L600 (94.5031, -48.8967) -> (94.404, -48.8459)
  line L601 (94.7571, -48.8459) -> (94.8561, -48.7951)
  line L602 (95.1584, -49.3997) -> (95.1076, -49.4505)
  line L603 (94.8561, -49.5013) -> (94.7571, -49.4505)
  line L604 (94.2008, -49.3997) -> (94.3024, -49.4505)
  line L605 (94.3024, -49.4505) -> (94.404, -49.4505)
  line L606 (95.0085, -49.5013) -> (94.8561, -49.5013)
  line L607 (95.2092, -49.2498) -> (95.1584, -49.3997)
  line L608 (94.15, -49.2498) -> (94.2008, -49.3997)
  line L609 (94.5031, -49.3997) -> (94.5539, -49.2981)
  line L610 (95.1076, -48.8459) -> (95.1584, -48.8967)
  line L611 (95.0085, -48.7951) -> (95.1076, -48.8459)
  line L612 (94.6555, -49.3489) -> (94.6047, -49.199)
  line L613 (94.7571, -49.4505) -> (94.6555, -49.3489)
  line L614 (94.8561, -48.7951) -> (95.0085, -48.7951)
  line L615 (94.6555, -48.945) -> (94.7571, -48.8459)
  line L616 (94.5539, -49.2981) -> (94.6047, -49.0974)
  line L617 (95.1076, -49.4505) -> (95.0085, -49.5013)
  line L618 (94.6047, -49.199) -> (94.5539, -48.9958)
  line L619 (94.6047, -49.0974) -> (94.6555, -48.945)
  line L620 (94.404, -49.4505) -> (94.5031, -49.3997)
  line L621 (94.5539, -48.9958) -> (94.5031, -48.8967)
  line L622 (95.2092, -49.0466) -> (95.2092, -49.2498)
  line L623 (94.15, -49.0466) -> (94.15, -49.2498)
  line L624 (94.404, -48.8459) -> (94.3024, -48.8459)
  line L625 (94.2008, -48.8967) -> (94.15, -49.0466)
  line L626 (95.1584, -48.8967) -> (95.2092, -49.0466)
  line L627 (94.2008, -48.2998) -> (94.15, -48.2008)
  line L628 (94.2516, -47.8477) -> (94.3532, -47.7969)
  line L629 (94.15, -48.2008) -> (94.15, -47.9976)
  line L630 (94.2008, -47.896) -> (94.2516, -47.8477)
  line L631 (94.15, -47.9976) -> (94.2008, -47.896)
  line L632 (94.2516, -48.3506) -> (94.2008, -48.2998)
  line L633 (94.3532, -47.7969) -> (94.4523, -47.7969)
  line L634 (94.4523, -47.7969) -> (94.5539, -47.8477)
  line L635 (94.404, -48.4014) -> (94.3532, -48.4014)
  line L636 (94.3532, -48.4014) -> (94.2516, -48.3506)
  line L637 (94.7063, -47.9468) -> (95.2092, -48.4522)
  line L638 (94.5539, -47.8477) -> (94.7063, -47.9468)
  line L639 (95.2092, -48.4522) -> (95.2092, -47.7461)
  line L640 (94.7571, -47.2508) -> (94.6555, -47.3524)
  line L641 (95.1584, -47.3016) -> (95.0593, -47.3524)
  line L642 (94.6555, -47.3524) -> (94.5031, -47.4032)
  line L643 (94.8053, -47.0502) -> (94.8053, -47.101)
  line L644 (94.8053, -47.101) -> (94.7571, -47.2508)
  line L645 (94.4523, -47.4032) -> (94.3024, -47.3524)
  line L646 (94.15, -47.0502) -> (94.2008, -46.8978)
  line L647 (95.2092, -47.0502) -> (95.2092, -47.1518)
  line L648 (94.15, -47.101) -> (94.15, -47.0502)
  line L649 (94.6555, -46.7987) -> (94.7571, -46.8978)
  line L650 (94.5031, -47.4032) -> (94.4523, -47.4032)
  line L651 (95.1584, -46.8978) -> (95.2092, -47.0502)
  line L652 (94.2008, -47.2508) -> (94.15, -47.101)
  line L653 (94.3024, -46.7987) -> (94.5031, -46.7479)
  line L654 (94.7571, -46.7479) -> (95.0085, -46.7987)
  line L655 (95.0085, -46.7987) -> (95.1584, -46.8978)
  line L656 (94.3024, -47.3524) -> (94.2008, -47.2508)
  line L657 (94.5031, -46.7479) -> (94.7571, -46.7479)
  line L658 (94.2008, -46.8978) -> (94.3024, -46.7987)
  line L659 (94.5031, -46.7479) -> (94.6555, -46.7987)
  line L660 (95.2092, -47.1518) -> (95.1584, -47.3016)
  line L661 (94.7571, -46.8978) -> (94.8053, -47.0502)
  line L662 (94.5031, -46.405) -> (95.2092, -46.405)
  line L663 (94.5539, -46.2526) -> (94.5031, -46.1535)
  line L664 (94.7063, -46.405) -> (94.5539, -46.2526)
  line L665 (94.7063, -45.8487) -> (95.2092, -45.8487)
  line L666 (94.5031, -46.1535) -> (94.5031, -46.0011)
  line L667 (94.5031, -46.0011) -> (94.5539, -45.8995)
  line L668 (94.5539, -45.8995) -> (94.7063, -45.8487)
  line L669 (94.5031, -45.5973) -> (94.5031, -45.4474)
  line L670 (94.7063, -45.8487) -> (94.5539, -45.6989)
  line L671 (94.5539, -45.3458) -> (94.7063, -45.295)
  line L672 (94.5031, -45.4474) -> (94.5539, -45.3458)
  line L673 (94.7063, -45.295) -> (95.2092, -45.295)
  line L674 (94.5539, -45.6989) -> (94.5031, -45.5973)
  line L675 (94.1018, -44.9013) -> (94.15, -44.9521)
  line L676 (94.15, -44.9521) -> (94.2008, -44.9013)
  line L677 (94.2008, -44.9013) -> (94.15, -44.8505)
  line L678 (94.15, -44.8505) -> (94.1018, -44.9013)
  line L679 (94.5031, -44.9013) -> (95.2092, -44.9013)
  line L680 (94.15, -44.5076) -> (95.2092, -44.5076)
  line L681 (90.1702, 37.2111) -> (98.1531, 37.2111)
  line L682 (90.1702, -135.7589) -> (98.1531, -135.7589)
  line L683 (95.6131, 37.2111) -> (95.8103, 36.475)
  line L684 (95.6131, 37.2111) -> (95.4158, 36.475)
  line L685 (95.6131, -135.7589) -> (95.8103, -135.0229)
  line L686 (95.6131, -135.7589) -> (95.4158, -135.0229)
  line L687 (95.6131, 37.2111) -> (95.6131, -44.4568)
  line L688 (95.6131, -54.091) -> (95.6131, -135.7589)
  line L689 (63.2462, 27.94) -> (63.2755, -25.4)
  line L690 (86.3601, 27.94) -> (63.2462, 27.94)
  line L691 (63.2755, -25.4) -> (86.3601, -25.4)
  line L692 (86.3601, -25.4) -> (86.3601, 27.94)
  line L693 (86.3601, 27.94) -> (86.3601, -15.24)
  line L694 (63.5002, -15.24) -> (63.5002, 26.67)
  line L695 (63.5002, 26.67) -> (64.7702, 27.94)
  line L696 (64.7702, 27.94) -> (86.3601, 27.94)
  line L697 (71.1201, 17.78) -> (71.1201, 27.94)
  line L698 (78.7402, 17.78) -> (71.1201, 17.78)
  line L699 (78.7402, 27.94) -> (78.7402, 17.78)
  line L700 (71.1201, 27.94) -> (78.7402, 27.94)
  line L701 (86.3601, -25.4) -> (63.5002, -25.4)
  line L702 (86.3601, 27.94) -> (63.2462, 27.94)
  line L703 (86.3601, -25.4) -> (86.3601, 27.94)
  line L704 (63.2462, 27.94) -> (63.2755, -25.4)
  line L705 (63.2755, -25.4) -> (86.3601, -25.4)
  line L706 (86.3601, 27.94) -> (86.3601, -15.24)
  line L707 (64.7702, 27.94) -> (86.3601, 27.94)
  line L708 (63.5002, 26.67) -> (64.7702, 27.94)
  line L709 (63.5002, -15.24) -> (63.5002, 26.67)
  line L710 (71.1201, 17.78) -> (71.1201, 27.94)
  line L711 (78.7402, 27.94) -> (78.7402, 17.78)
  line L712 (78.7402, 17.78) -> (71.1201, 17.78)
  line L713 (71.1201, 27.94) -> (78.7402, 27.94)
  line L714 (86.3601, -25.4) -> (63.5002, -25.4)
  line L715 (65.7437, 24.9955) -> (65.5621, 25.2455)
  line L716 (66.0376, 24.9001) -> (65.7437, 24.9955)
  line L717 (66.3366, 24.9955) -> (66.0427, 24.9001)
  line L718 (65.5621, 25.5546) -> (65.7437, 25.8046)
  line L719 (66.0427, 24.9001) -> (66.0376, 24.9001)
  line L720 (65.5621, 25.2455) -> (65.5621, 25.5546)
  line L721 (66.0376, 25.9001) -> (66.0427, 25.9001)
  line L722 (66.5182, 25.5546) -> (66.5182, 25.2455)
  line L723 (66.3366, 25.8046) -> (66.5182, 25.5546)
  line L724 (66.5182, 25.2455) -> (66.3366, 24.9955)
  line L725 (66.0427, 25.9001) -> (66.3366, 25.8046)
  line L726 (65.7437, 25.8046) -> (66.0376, 25.9001)
  line L727 (65.7437, 23.2646) -> (66.0376, 23.36)
  line L728 (66.5182, 22.7055) -> (66.3366, 22.4555)
  line L729 (65.7437, 22.4555) -> (65.5621, 22.7055)
  line L730 (66.3366, 22.4555) -> (66.0427, 22.36)
  line L731 (65.5621, 22.7055) -> (65.5621, 23.0146)
  line L732 (65.5621, 23.0146) -> (65.7437, 23.2646)
  line L733 (66.3366, 23.2646) -> (66.5182, 23.0146)
  line L734 (66.0376, 23.36) -> (66.0427, 23.36)
  line L735 (66.5182, 23.0146) -> (66.5182, 22.7055)
  line L736 (66.0427, 23.36) -> (66.3366, 23.2646)
  line L737 (66.0427, 22.36) -> (66.0376, 22.36)
  line L738 (66.0376, 22.36) -> (65.7437, 22.4555)
  line L739 (65.7437, 19.9155) -> (65.5621, 20.1655)
  line L740 (65.5621, 20.4745) -> (65.7437, 20.7245)
  line L741 (66.3366, 19.9155) -> (66.0427, 19.82)
  line L742 (66.0376, 20.82) -> (66.0427, 20.82)
  line L743 (66.0427, 19.82) -> (66.0376, 19.82)
  line L744 (66.5182, 20.1655) -> (66.3366, 19.9155)
  line L745 (65.7437, 20.7245) -> (66.0376, 20.82)
  line L746 (66.0427, 20.82) -> (66.3366, 20.7245)
  line L747 (65.5621, 20.1655) -> (65.5621, 20.4745)
  line L748 (66.0376, 19.82) -> (65.7437, 19.9155)
  line L749 (66.5182, 20.4745) -> (66.5182, 20.1655)
  line L750 (66.3366, 20.7245) -> (66.5182, 20.4745)
  line L751 (65.5621, 17.9345) -> (65.7437, 18.1845)
  line L752 (65.7437, 17.3755) -> (65.5621, 17.6255)
  line L753 (66.0376, 18.28) -> (66.0427, 18.28)
  line L754 (66.5182, 17.9345) -> (66.5182, 17.6255)
  line L755 (66.0376, 17.28) -> (65.7437, 17.3755)
  line L756 (66.0427, 18.28) -> (66.3366, 18.1845)
  line L757 (66.3366, 17.3755) -> (66.0427, 17.28)
  line L758 (65.5621, 17.6255) -> (65.5621, 17.9345)
  line L759 (66.3366, 18.1845) -> (66.5182, 17.9345)
  line L760 (65.7437, 18.1845) -> (66.0376, 18.28)
  line L761 (66.5182, 17.6255) -> (66.3366, 17.3755)
  line L762 (66.0427, 17.28) -> (66.0376, 17.28)
  line L763 (66.0376, 15.74) -> (66.0427, 15.74)
  line L764 (66.3366, 15.6445) -> (66.5182, 15.3945)
  line L765 (66.0376, 14.74) -> (65.7437, 14.8355)
  line L766 (66.5182, 15.3945) -> (66.5182, 15.0855)
  line L767 (65.7437, 14.8355) -> (65.5621, 15.0855)
  line L768 (65.5621, 15.0855) -> (65.5621, 15.3945)
  line L769 (66.0427, 14.74) -> (66.0376, 14.74)
  line L770 (66.3366, 14.8355) -> (66.0427, 14.74)
  line L771 (66.5182, 15.0855) -> (66.3366, 14.8355)
  line L772 (65.5621, 15.3945) -> (65.7437, 15.6445)
  line L773 (66.0427, 15.74) -> (66.3366, 15.6445)
  line L774 (65.7437, 15.6445) -> (66.0376, 15.74)
  line L775 (66.3366, 13.1045) -> (66.5182, 12.8545)
  line L776 (66.0427, 13.2) -> (66.3366, 13.1045)
  line L777 (65.5621, 12.5455) -> (65.5621, 12.8545)
  line L778 (66.5182, 12.8545) -> (66.5182, 12.5455)
  line L779 (66.0427, 12.2) -> (66.0376, 12.2)
  line L780 (65.7437, 12.2955) -> (65.5621, 12.5455)
  line L781 (66.5182, 12.5455) -> (66.3366, 12.2955)
  line L782 (66.0376, 13.2) -> (66.0427, 13.2)
  line L783 (65.5621, 12.8545) -> (65.7437, 13.1045)
  line L784 (66.3366, 12.2955) -> (66.0427, 12.2)
  line L785 (65.7437, 13.1045) -> (66.0376, 13.2)
  line L786 (66.0376, 12.2) -> (65.7437, 12.2955)
  line L787 (66.3366, 9.7555) -> (66.0427, 9.66)
  line L788 (66.0376, 9.66) -> (65.7437, 9.7555)
  line L789 (65.7437, 10.5645) -> (66.0376, 10.66)
  line L790 (66.3366, 10.5645) -> (66.5182, 10.3145)
  line L791 (65.5621, 10.0055) -> (65.5621, 10.3145)
  line L792 (66.0376, 10.66) -> (66.0427, 10.66)
  line L793 (65.7437, 9.7555) -> (65.5621, 10.0055)
  line L794 (66.0427, 9.66) -> (66.0376, 9.66)
  line L795 (66.0427, 10.66) -> (66.3366, 10.5645)
  line L796 (66.5182, 10.0055) -> (66.3366, 9.7555)
  line L797 (65.5621, 10.3145) -> (65.7437, 10.5645)
  line L798 (66.5182, 10.3145) -> (66.5182, 10.0055)
  line L799 (65.5621, 7.4655) -> (65.5621, 7.7745)
  line L800 (66.3366, 7.2155) -> (66.0427, 7.12)
  line L801 (66.0427, 7.12) -> (66.0376, 7.12)
  line L802 (66.0376, 7.12) -> (65.7437, 7.2155)
  line L803 (65.7437, 7.2155) -> (65.5621, 7.4655)
  line L804 (66.5182, 7.7745) -> (66.5182, 7.4655)
  line L805 (65.5621, 7.7745) -> (65.7437, 8.0245)
  line L806 (66.5182, 7.4655) -> (66.3366, 7.2155)
  line L807 (65.7437, 8.0245) -> (66.0376, 8.12)
  line L808 (66.3366, 8.0245) -> (66.5182, 7.7745)
  line L809 (66.0427, 8.12) -> (66.3366, 8.0245)
  line L810 (66.0376, 8.12) -> (66.0427, 8.12)
  line L811 (66.5182, 4.9255) -> (66.3366, 4.6755)
  line L812 (66.0427, 4.58) -> (66.0376, 4.58)
  line L813 (66.5182, 5.2345) -> (66.5182, 4.9255)
  line L814 (65.7437, 5.4845) -> (66.0376, 5.58)
  line L815 (65.7437, 4.6755) -> (65.5621, 4.9255)
  line L816 (66.3366, 5.4845) -> (66.5182, 5.2345)
  line L817 (66.0376, 4.58) -> (65.7437, 4.6755)
  line L818 (66.0427, 5.58) -> (66.3366, 5.4845)
  line L819 (66.0376, 5.58) -> (66.0427, 5.58)
  line L820 (66.3366, 4.6755) -> (66.0427, 4.58)
  line L821 (65.5621, 5.2345) -> (65.7437, 5.4845)
  line L822 (65.5621, 4.9255) -> (65.5621, 5.2345)
  line L823 (65.7437, 2.1355) -> (65.5621, 2.3855)
  line L824 (66.0427, 3.04) -> (66.3366, 2.9445)
  line L825 (66.5182, 2.6945) -> (66.5182, 2.3855)
  line L826 (65.7437, 2.9445) -> (66.0376, 3.04)
  line L827 (66.3366, 2.1355) -> (66.0427, 2.04)
  line L828 (65.5621, 2.6945) -> (65.7437, 2.9445)
  line L829 (66.0427, 2.04) -> (66.0376, 2.04)
  line L830 (66.3366, 2.9445) -> (66.5182, 2.6945)
  line L831 (65.5621, 2.3855) -> (65.5621, 2.6945)
  line L832 (66.0376, 3.04) -> (66.0427, 3.04)
  line L833 (66.5182, 2.3855) -> (66.3366, 2.1355)
  line L834 (66.0376, 2.04) -> (65.7437, 2.1355)
  line L835 (65.5621, -0.1545) -> (65.5621, 0.1545)
  line L836 (66.0376, -0.5) -> (65.7437, -0.4045)
  line L837 (66.0427, 0.5) -> (66.3366, 0.4045)
  line L838 (66.0376, 0.5) -> (66.0427, 0.5)
  line L839 (65.7437, 0.4045) -> (66.0376, 0.5)
  line L840 (65.5621, 0.1545) -> (65.7437, 0.4045)
  line L841 (66.5182, -0.1545) -> (66.3366, -0.4045)
  line L842 (66.3366, 0.4045) -> (66.5182, 0.1545)
  line L843 (65.7437, -0.4045) -> (65.5621, -0.1545)
  line L844 (66.5182, 0.1545) -> (66.5182, -0.1545)
  line L845 (66.3366, -0.4045) -> (66.0427, -0.5)
  line L846 (66.0427, -0.5) -> (66.0376, -0.5)
  line L847 (65.5621, -2.6945) -> (65.5621, -2.3855)
  line L848 (66.0376, -3.04) -> (65.7437, -2.9445)
  line L849 (66.5182, -2.6945) -> (66.3366, -2.9445)
  line L850 (65.7437, -2.9445) -> (65.5621, -2.6945)
  line L851 (66.3366, -2.9445) -> (66.0427, -3.04)
  line L852 (66.0427, -2.04) -> (66.3366, -2.1355)
  line L853 (65.5621, -2.3855) -> (65.7437, -2.1355)
  line L854 (66.5182, -2.3855) -> (66.5182, -2.6945)
  line L855 (66.3366, -2.1355) -> (66.5182, -2.3855)
  line L856 (66.0427, -3.04) -> (66.0376, -3.04)
  line L857 (65.7437, -2.1355) -> (66.0376, -2.04)
  line L858 (66.0376, -2.04) -> (66.0427, -2.04)
  line L859 (66.3366, -4.6755) -> (66.5182, -4.9255)
  line L860 (66.0427, -5.58) -> (66.0376, -5.58)
  line L861 (66.0376, -4.58) -> (66.0427, -4.58)
  line L862 (66.3366, -5.4845) -> (66.0427, -5.58)
  line L863 (66.0427, -4.58) -> (66.3366, -4.6755)
  line L864 (66.5182, -4.9255) -> (66.5182, -5.2345)
  line L865 (65.5621, -4.9255) -> (65.7437, -4.6755)
  line L866 (65.7437, -4.6755) -> (66.0376, -4.58)
  line L867 (66.5182, -5.2345) -> (66.3366, -5.4845)
  line L868 (65.5621, -5.2345) -> (65.5621, -4.9255)
  line L869 (65.7437, -5.4845) -> (65.5621, -5.2345)
  line L870 (66.0376, -5.58) -> (65.7437, -5.4845)
  line L871 (65.7437, -7.2155) -> (66.0376, -7.12)
  line L872 (65.5621, -7.7745) -> (65.5621, -7.4655)
  line L873 (66.5182, -7.7745) -> (66.3366, -8.0245)
  line L874 (66.3366, -7.2155) -> (66.5182, -7.4655)
  line L875 (66.0376, -7.12) -> (66.0427, -7.12)
  line L876 (65.7437, -8.0245) -> (65.5621, -7.7745)
  line L877 (65.5621, -7.4655) -> (65.7437, -7.2155)
  line L878 (66.0427, -7.12) -> (66.3366, -7.2155)
  line L879 (66.5182, -7.4655) -> (66.5182, -7.7745)
  line L880 (66.0427, -8.12) -> (66.0376, -8.12)
  line L881 (66.3366, -8.0245) -> (66.0427, -8.12)
  line L882 (66.0376, -8.12) -> (65.7437, -8.0245)
  line L883 (66.3366, -9.7555) -> (66.5182, -10.0055)
  line L884 (66.0376, -10.66) -> (65.7437, -10.5645)
  line L885 (66.3366, -10.5645) -> (66.0427, -10.66)
  line L886 (65.7437, -9.7555) -> (66.0376, -9.66)
  line L887 (65.5621, -10.0055) -> (65.7437, -9.7555)
  line L888 (66.0427, -10.66) -> (66.0376, -10.66)
  line L889 (66.0427, -9.66) -> (66.3366, -9.7555)
  line L890 (66.5182, -10.0055) -> (66.5182, -10.3145)
  line L891 (65.7437, -10.5645) -> (65.5621, -10.3145)
  line L892 (65.5621, -10.3145) -> (65.5621, -10.0055)
  line L893 (66.0376, -9.66) -> (66.0427, -9.66)
  line L894 (66.5182, -10.3145) -> (66.3366, -10.5645)
  line L895 (66.0427, -13.2) -> (66.0376, -13.2)
  line L896 (66.5182, -12.8545) -> (66.3366, -13.1045)
  line L897 (66.0427, -12.2) -> (66.3366, -12.2955)
  line L898 (66.3366, -12.2955) -> (66.5182, -12.5455)
  line L899 (65.7437, -12.2955) -> (66.0376, -12.2)
  line L900 (65.5621, -12.8545) -> (65.5621, -12.5455)
  line L901 (65.5621, -12.5455) -> (65.7437, -12.2955)
  line L902 (66.0376, -12.2) -> (66.0427, -12.2)
  line L903 (66.0376, -13.2) -> (65.7437, -13.1045)
  line L904 (66.5182, -12.5455) -> (66.5182, -12.8545)
  line L905 (66.3366, -13.1045) -> (66.0427, -13.2)
  line L906 (65.7437, -13.1045) -> (65.5621, -12.8545)
  line L907 (66.3292, -15.6407) -> (66.0353, -15.7362)
  line L908 (66.0302, -14.7362) -> (66.0353, -14.7362)
  line L909 (65.7363, -14.8317) -> (66.0302, -14.7362)
  line L910 (65.7363, -15.6407) -> (65.5547, -15.3907)
  line L911 (66.5108, -15.0817) -> (66.5108, -15.3907)
  line L912 (66.3292, -14.8317) -> (66.5108, -15.0817)
  line L913 (65.5547, -15.3907) -> (65.5547, -15.0817)
  line L914 (66.0353, -15.7362) -> (66.0302, -15.7362)
  line L915 (66.5108, -15.3907) -> (66.3292, -15.6407)
  line L916 (66.0302, -15.7362) -> (65.7363, -15.6407)
  line L917 (66.0353, -14.7362) -> (66.3292, -14.8317)
  line L918 (65.5547, -15.0817) -> (65.7363, -14.8317)
  line L919 (65.7437, -18.1845) -> (65.5621, -17.9345)
  line L920 (65.5621, -17.9345) -> (65.5621, -17.6255)
  line L921 (66.0427, -17.28) -> (66.3366, -17.3755)
  line L922 (66.5182, -17.6255) -> (66.5182, -17.9345)
  line L923 (65.7437, -17.3755) -> (66.0376, -17.28)
  line L924 (66.0376, -17.28) -> (66.0427, -17.28)
  line L925 (66.0376, -18.28) -> (65.7437, -18.1845)
  line L926 (65.5621, -17.6255) -> (65.7437, -17.3755)
  line L927 (66.5182, -17.9345) -> (66.3366, -18.1845)
  line L928 (66.3366, -18.1845) -> (66.0427, -18.28)
  line L929 (66.0427, -18.28) -> (66.0376, -18.28)
  line L930 (66.3366, -17.3755) -> (66.5182, -17.6255)
  line L931 (66.3366, -20.7245) -> (66.0427, -20.82)
  line L932 (66.0376, -19.82) -> (66.0427, -19.82)
  line L933 (66.3366, -19.9155) -> (66.5182, -20.1655)